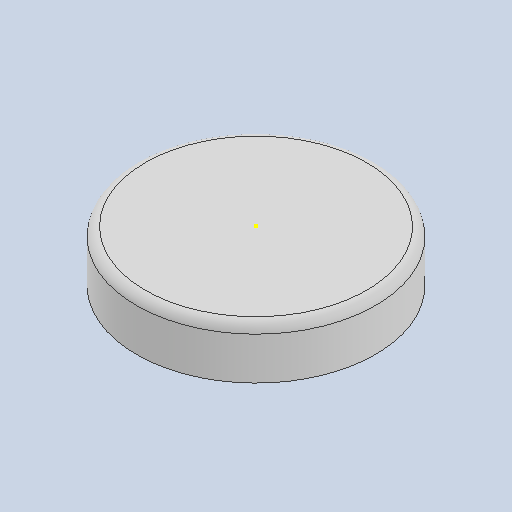
# Autodesk Inventor part: Drehplatform_prototyp
Saved by Autodesk Inventor 2023 (Build 270158000, 158)
## iProperties
Created: 2022-06-11
Part Number: Drehplatform_prototyp
Material: Generic
Document SubType Name: Modeling
Designer: Habib
Density: 1 g/cm^3
Appearance: Default
Author: Habib
Autodesk Inventor part; units mm, degrees
ref_plane "YZ Plane" through (0, 0, 0) normal (1, 0, 0) x (0, 1, 0)
ref_plane "XZ Plane" through (0, 0, 0) normal (0, 1, 0) x (-1, 0, 0)
ref_plane "XY Plane" through (0, 0, 0) normal (0, 0, 1) x (1, 0, 0)
sketch "Sketch1" plane through (0, 0, 0) normal (0, 1, 0) x (-1, 0, 0)
  circle A0 centre (0, 0) radius 70
  dimension "d0" = 140
  constraints: 1 centre point, 1 coincident
  measures "d0" diameter of A0
extrude "Extrusion1" add sketch "Sketch1" along normal blind 30
sketch "Sketch2" plane through (0, 30, 0) normal (0, 1, 0) x (1, 0, 0)
  point P0 (0, 0)
fillet "Fillet1" radius 5.175 1 edges at (70, 30, 0)
sketch "Sketch3" plane through (0, 0, 0) normal (0, -1, 0) x (1, 0, 0)
  circle A0 centre (0, 0) radius 65
  dimension "d4" = 130
  constraints: 1 centre point, 1 coincident
  measures "d4" diameter of A0
extrude "Extrusion2" cut sketch "Sketch3" against normal blind 25
sketch "Sketch5" plane through (0, 25, 0) normal (0, -1, 0) x (1, 0, 0)
  line L0 (-7, 0) -> (7, 0) construction
  line L1 (-7, -3) -> (7, -3)
  line L2 (7, 3) -> (-7, 3)
  arc A0 (-7, 3) -> (-7, -3) centre (-7, 0) ccw
  arc A1 (7, -3) -> (7, 3) centre (7, 0) ccw
  point P0 (0, 0)
  dimension "d11" = 7
  dimension "d12" = 6
  constraints: 8 end point, 4 point on circle, 4 tangent, 2 centre point, 1 horizontal, 1 midpoint, 1 parallel
  measures "d11" distance of point (0, 0) L0.end
  measures "d12" diameter of A1
extrude "Extrusion4" add sketch "Sketch5" along normal blind 20
sketch "Sketch6" plane through (0, 5, 0) normal (0, -1, 0) x (1, 0, 0)
  line L0 (-5, 0) -> (5, 0) construction
  line L1 (-5, -1.5) -> (5, -1.5)
  line L2 (5, 1.5) -> (-5, 1.5)
  arc A0 (-5, 1.5) -> (-5, -1.5) centre (-5, 0) ccw
  arc A1 (5, -1.5) -> (5, 1.5) centre (5, 0) ccw
  point P0 (0, 0)
  dimension "d15" = 5
  dimension "d16" = 3
  constraints: 8 end point, 4 point on circle, 4 tangent, 2 centre point, 1 horizontal, 1 midpoint, 1 parallel
  measures "d15" distance of point (0, 0) L0.end
  measures "d16" diameter of A1
extrude "Extrusion5" cut sketch "Sketch6" against normal blind 20
body "Solid1"
